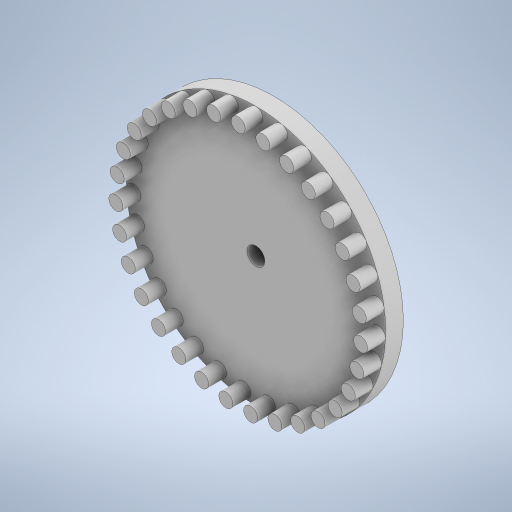
# Autodesk Inventor part: 사이클로이드 기어 002
Saved by Autodesk Inventor 2023 (Build 270158000, 158)
## iProperties
Created: 2022-06-19
Part Number: 사이클로이드 기어 002
Material: 일반
Document SubType Name: Modeling
Designer: fly01
Density: 1 g/cm^3
Appearance: 기본값
Author: fly01
Autodesk Inventor part; units mm, degrees
ref_plane "YZ Plane" through (0, 0, 0) normal (1, 0, 0) x (0, 1, 0)
ref_plane "XZ Plane" through (0, 0, 0) normal (0, 1, 0) x (-1, 0, 0)
ref_plane "XY Plane" through (0, 0, 0) normal (0, 0, 1) x (1, 0, 0)
sketch "스케치1" plane through (0, 0, 0) normal (0, 0, 1) x (1, 0, 0)
  circle A0 centre (0, 0) radius 32.5
  circle A1 centre (0, 34.5) radius 2
  circle A2 centre (0, 0) radius 36.5
  dimension "d0" = 65
  dimension "d1" = 4
  dimension "d2" = 73
  constraints: 3 centre point, 2 coincident, 1 tangent
  measures "d0" diameter of A0
  measures "d1" diameter of A1
  measures "d2" diameter of A2
extrude "돌출1" add sketch "스케치1" against normal blind 5 contours A0 | A2 | A1
extrude "돌출2" add sketch "스케치1" along normal blind 5 contours A1
pattern_circular "원형 패턴1" count 31 over 360 about axis through (0, 0, 0) along (0, 0, -1) of "돌출2"
sketch "스케치2" plane through (0, 0, 0) normal (0, 0, 1) x (1, 0, 0)
  circle A0 centre (0, 0) radius 2.5
  dimension "d10" = 5
  constraints: 1 centre point, 1 coincident
  measures "d10" diameter of A0
extrude "돌출3" cut sketch "스케치2" against normal blind 5
